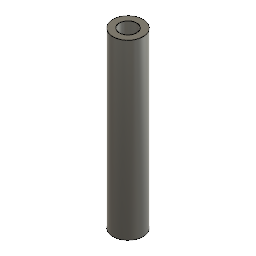
3d (Autodesk Fusion 360 archive; units mm, degrees)
design "mount_pole"
Autodesk Fusion 360 part; units mm, degrees
note: some values were not read from the file. Chosen so that the rebuilt part matches the saved one: which face or edge a step refers to.
sketch "Sketch1" plane through (0, 0, 0) normal (0, 1, 0) x (1, 0, 0)
  circle A0 centre (0, 0) radius 3.5
  circle A1 centre (0, 0) radius 2
  dimension "d1" = 7
  dimension "d2" = 4
  measures "d1" diameter of A0
  measures "d2" diameter of A1
extrude "Extrude1" add sketch "Sketch1" along normal blind 40

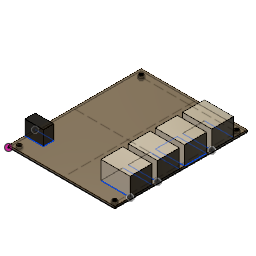
design "ZodiacFX"
Autodesk Fusion 360 part; units mm, degrees
sketch "Sketch1" plane through (0, 0, 0) normal (0, 1, 0) x (1, 0, 0)
  line L0 (0, 0) -> (80, 0)
  line L1 (80, 0) -> (80, 100)
  line L2 (80, 100) -> (0, 100)
  line L3 (0, 100) -> (0, 0)
  circle A0 centre (4, 96) radius 1.5
  circle A1 centre (76, 96) radius 1.5
  circle A2 centre (76, 4) radius 1.5
  circle A3 centre (4, 4) radius 1.5
  line L4 (40, 100) -> (40, 0) construction
  line L5 (0, 50) -> (80, 50) construction
  line L6 (4, 96) -> (40, 96) construction
  line L7 (76, 96) -> (76, 50) construction
  line L8 (76, 96) -> (40, 96) construction
  line L9 (76, 50) -> (76, 4) construction
  dimension "d1" = 80
  dimension "d2" = 100
  dimension "d3" = 3
  dimension "d4" = 72
  dimension "d5" = 92
  measures "d1" distance of L0.start
  measures "d3" diameter of A0
  measures "d5" distance of L0.start
extrude "Extrude1" add sketch "Sketch1" along normal blind 1.6
sketch "Sketch2" plane through (0, 1.6, 0) normal (0, 1, 0) x (-1, 0, 0)
  circle A0 centre (-4, -96) radius 1.5
  circle A1 centre (-4, -4) radius 1.5
  circle A2 centre (-76, -96) radius 1.5
  circle A3 centre (-76, -4) radius 1.5
  line L0 (0, -100) -> (0, 0)
  line L1 (0, 0) -> (-80, 0)
  line L2 (-80, 0) -> (-80, -100)
  line L3 (-80, -100) -> (0, -100)
  line L4 (-58, -89.6377) -> (-80, -89.6377)
  line L5 (-80, -89.6377) -> (-80, -73.1377)
  line L6 (-80, -73.1377) -> (-58, -73.1377)
  line L7 (-58, -73.1377) -> (-58, -89.6377)
  line L8 (-58, -69.1377) -> (-80, -69.1377)
  line L9 (-80, -69.1377) -> (-80, -52.6377)
  line L10 (-80, -52.6377) -> (-58, -52.6377)
  line L11 (-58, -52.6377) -> (-58, -69.1377)
  line L12 (-58, -48.6377) -> (-80, -48.6377)
  line L13 (-80, -48.6377) -> (-80, -32.1377)
  line L14 (-80, -32.1377) -> (-58, -32.1377)
  line L15 (-58, -32.1377) -> (-58, -48.6377)
  line L16 (-58, -28.1377) -> (-80, -28.1377)
  line L17 (-80, -28.1377) -> (-80, -11.6377)
  line L18 (-80, -11.6377) -> (-58, -11.6377)
  line L19 (-58, -11.6377) -> (-58, -28.1377)
  line L20 (0, -20) -> (-14.1052, -20)
  line L21 (-14.1052, -20) -> (-14.1052, -12.0995)
  line L22 (-14.1052, -12.0995) -> (0, -12.0995)
  line L23 (0, -12.0995) -> (0, -20)
  dimension "d8" = 16.5
  dimension "d9" = 22
  dimension "d10" = 4
  dimension "d11" = 4
  dimension "d12" = 4
  measures "d10" distance of L6 L8
  measures "d11" distance of L10 L12
  measures "d12" distance of L14 L16
extrude "Extrude2" add sketch "Sketch2" along normal blind 13.8 contours L2 L4 L5 L6 L7 | L2 L8 L9 L10 L11 | L2 L16 L17 L18 L19 | L2 L12 L13 L14 L15
extrude "Extrude3" add sketch "Sketch2" along normal blind 11 contours L0 L20 L21 L22 L23
sketch "Sketch3" plane through (0, 1.6, 0) normal (0, 1, 0) x (-1, 0, 0)

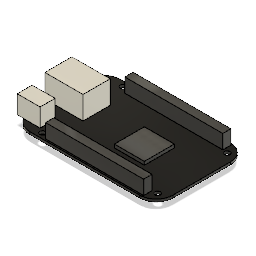
design "BeagleBoneBlack"
Autodesk Fusion 360 part; units mm, degrees
sketch "Sketch1" plane through (0, 0, 0) normal (0, 1, 0) x (1, 0, 0)
  line L0 (10, 0) -> (76.2, 0)
  line L1 (86.2, 10) -> (86.2, 44.61)
  line L2 (76.2, 54.61) -> (10, 54.61)
  line L3 (0, 44.61) -> (0, 10)
  circle A0 centre (14.6, 51.435) radius 1.6
  circle A1 centre (14.6, 3.175) radius 1.6
  circle A2 centre (80.64, 48.26) radius 1.6
  circle A3 centre (80.64, 6.35) radius 1.6
  arc A4 (0, 10) -> (10, 0) centre (10, 10) ccw
  arc A5 (10, 54.61) -> (0, 44.61) centre (10, 44.61) ccw
  arc A6 (86.2, 44.61) -> (76.2, 54.61) centre (76.2, 44.61) ccw
  arc A7 (76.2, 0) -> (86.2, 10) centre (76.2, 10) ccw
  dimension "d1" = 86.2
  dimension "d2" = 54.61
  dimension "d3" = 3.2
  dimension "d4" = 14.6
  dimension "d5" = 3.175
  dimension "d6" = 48.26
  dimension "d8" = 41.91
  dimension "d10" = 6.35
  dimension "d11" = 65.9
  dimension "d12" = 66.04
  dimension "d13" = 10
  dimension "d36" = 3.11
  measures "d1" distance of origin
  measures "d2" distance of origin
  measures "d3" diameter of A1
  measures "d4" distance of L3
  measures "d5" distance of L2
  measures "d8" distance of origin
  measures "d10" distance of L0
  measures "d12" distance of origin
  measures "d13" radius of A4
extrude "Extrude1" add sketch "Sketch1" along normal blind 1.6
sketch "Sketch2" plane through (0, 1.6, 0) normal (0, 1, 0) x (-1, 0, 0)
  circle A0 centre (-14.6, -3.175) radius 1.6
  circle A1 centre (-80.64, -6.35) radius 1.6
  circle A2 centre (-14.6, -51.435) radius 1.6
  circle A3 centre (-80.64, -48.26) radius 1.6
  arc A4 (-76.2, 0) -> (-86.2, -10) centre (-76.2, -10) ccw
  line L0 (-86.2, -10) -> (-86.2, -44.61)
  arc A5 (-86.2, -44.61) -> (-76.2, -54.61) centre (-76.2, -44.61) ccw
  line L1 (-76.2, -54.61) -> (-10, -54.61)
  arc A6 (-10, -54.61) -> (0, -44.61) centre (-10, -44.61) ccw
  line L2 (0, -44.61) -> (0, -10)
  arc A7 (0, -10) -> (-10, 0) centre (-10, -10) ccw
  line L3 (-10, 0) -> (-76.2, 0)
  line L4 (-18.553, -6) -> (-77.553, -6)
  line L5 (-77.553, -6) -> (-77.553, -1)
  line L6 (-77.553, -1) -> (-18.553, -1)
  line L7 (-18.553, -1) -> (-18.553, -6)
  line L8 (-18.553, -53.61) -> (-77.553, -53.61)
  line L9 (-77.553, -53.61) -> (-77.553, -48.61)
  line L10 (-77.553, -48.61) -> (-18.553, -48.61)
  line L11 (-18.553, -48.61) -> (-18.553, -53.61)
  dimension "d16" = 59
  dimension "d17" = 1
  dimension "d18" = 1
  dimension "d19" = 5
  measures "d16" distance of origin
  measures "d17" distance of L1 L8
  measures "d18" distance of L3 L6
extrude "Extrude2" add sketch "Sketch2" along normal blind 8.5 contours L4 L5 L6 L7 | L8 L9 L10 L11
sketch "Sketch3" plane through (0, 1.6, 0) normal (0, 1, 0) x (-1, 0, 0)
  line L0 (-18.553, -1) -> (-18.553, -6)
  line L1 (-18.553, -6) -> (-77.553, -6)
  line L2 (-77.553, -6) -> (-77.553, -1)
  line L3 (-77.553, -1) -> (-18.553, -1)
  line L4 (-18.553, -48.61) -> (-18.553, -53.61)
  line L5 (-18.553, -53.61) -> (-77.553, -53.61)
  line L6 (-77.553, -53.61) -> (-77.553, -48.61)
  line L7 (-77.553, -48.61) -> (-18.553, -48.61)
  circle A0 centre (-14.6, -3.175) radius 1.6
  circle A1 centre (-80.64, -6.35) radius 1.6
  circle A2 centre (-14.6, -51.435) radius 1.6
  circle A3 centre (-80.64, -48.26) radius 1.6
  arc A4 (-76.2, 0) -> (-86.2, -10) centre (-76.2, -10) ccw
  line L8 (-86.2, -10) -> (-86.2, -44.61)
  arc A5 (-86.2, -44.61) -> (-76.2, -54.61) centre (-76.2, -44.61) ccw
  line L9 (-76.2, -54.61) -> (-10, -54.61)
  arc A6 (-10, -54.61) -> (0, -44.61) centre (-10, -44.61) ccw
  line L10 (0, -44.61) -> (0, -10)
  arc A7 (0, -10) -> (-10, 0) centre (-10, -10) ccw
  line L11 (-10, 0) -> (-76.2, 0)
  line L12 (2.5, -37.91) -> (-20.5, -37.91)
  line L13 (-20.5, -37.91) -> (-20.5, -21.61)
  line L14 (-20.5, -21.61) -> (2.5, -21.61)
  line L15 (2.5, -21.61) -> (2.5, -37.91)
  dimension "d22" = 16.3
  dimension "d23" = 16.7
  dimension "d24" = 2.5
  measures "d23" distance of L9 L12
  measures "d24" distance of L10 L15
extrude "Extrude3" add sketch "Sketch3" along normal blind 13.8 contours L10 L12 L14 L15 | L10 L12 L13 L14
sketch "Sketch4" plane through (0, 1.6, 0) normal (0, 1, 0) x (-1, 0, 0)
  line L0 (-20.5, -21.61) -> (0, -21.61)
  line L1 (0, -21.61) -> (0, -10)
  arc A0 (0, -10) -> (-10, 0) centre (-10, -10) ccw
  line L2 (-10, 0) -> (-76.2, 0)
  arc A1 (-76.2, 0) -> (-86.2, -10) centre (-76.2, -10) ccw
  line L3 (-86.2, -10) -> (-86.2, -44.61)
  arc A2 (-86.2, -44.61) -> (-76.2, -54.61) centre (-76.2, -44.61) ccw
  line L4 (-76.2, -54.61) -> (-10, -54.61)
  arc A3 (-10, -54.61) -> (0, -44.61) centre (-10, -44.61) ccw
  line L5 (0, -44.61) -> (0, -37.91)
  line L6 (0, -37.91) -> (-20.5, -37.91)
  line L7 (-20.5, -37.91) -> (-20.5, -21.61)
  line L8 (-18.553, -1) -> (-18.553, -6)
  line L9 (-18.553, -6) -> (-77.553, -6)
  line L10 (-77.553, -6) -> (-77.553, -1)
  line L11 (-77.553, -1) -> (-18.553, -1)
  line L12 (-18.553, -48.61) -> (-18.553, -53.61)
  line L13 (-18.553, -53.61) -> (-77.553, -53.61)
  line L14 (-77.553, -53.61) -> (-77.553, -48.61)
  line L15 (-77.553, -48.61) -> (-18.553, -48.61)
  circle A4 centre (-14.6, -3.175) radius 1.6
  circle A5 centre (-80.64, -6.35) radius 1.6
  circle A6 centre (-14.6, -51.435) radius 1.6
  circle A7 centre (-80.64, -48.26) radius 1.6
  line L16 (2.5, -14) -> (-11.3258, -14)
  line L17 (-11.3258, -14) -> (-11.3258, -5)
  line L18 (-11.3258, -5) -> (2.5, -5)
  line L19 (2.5, -5) -> (2.5, -14)
  dimension "d27" = 9
  dimension "d28" = 5
  measures "d28" distance of L18
extrude "Extrude4" add sketch "Sketch4" along normal blind 11 contours L1 A0 L16 L17 L18 | L1 A0 L16 L18 L19
sketch "Sketch5" plane through (0, 0, 0) normal (0, -1, 0) x (1, 0, 0)
  circle A0 centre (14.6, -3.175) radius 1.6
  circle A1 centre (80.64, -6.35) radius 1.6
  circle A2 centre (14.6, -51.435) radius 1.6
  circle A3 centre (80.64, -48.26) radius 1.6
  arc A4 (86.2, -10) -> (76.2, 0) centre (76.2, -10) ccw
  line L0 (76.2, 0) -> (10, 0)
  arc A5 (10, 0) -> (0, -10) centre (10, -10) ccw
  line L1 (0, -10) -> (0, -44.61)
  arc A6 (0, -44.61) -> (10, -54.61) centre (10, -44.61) ccw
  line L2 (10, -54.61) -> (76.2, -54.61)
  arc A7 (76.2, -54.61) -> (86.2, -44.61) centre (76.2, -44.61) ccw
  line L3 (86.2, -44.61) -> (86.2, -10)
  line L4 (-0.5891, -40.4049) -> (7.6203, -40.4049)
  line L5 (7.6203, -40.4049) -> (7.6203, -46.4306)
  line L6 (7.6203, -46.4306) -> (-0.5891, -46.4306)
  line L7 (-0.5891, -46.4306) -> (-0.5891, -40.4049)
extrude "Extrude5" add sketch "Sketch5" along normal blind 3.9 contours L1 A6 L4 L5 L6 | L1 A6 L4 L6 L7
sketch "Sketch6" plane through (0, 1.6, 0) normal (0, 1, 0) x (-1, 0, 0)
  line L0 (-11.3258, -5) -> (-1.3397, -5)
  arc A0 (-1.3397, -5) -> (-10, 0) centre (-10, -10) ccw
  line L1 (-10, 0) -> (-76.2, 0)
  arc A1 (-76.2, 0) -> (-86.2, -10) centre (-76.2, -10) ccw
  line L2 (-86.2, -10) -> (-86.2, -44.61)
  arc A2 (-86.2, -44.61) -> (-76.2, -54.61) centre (-76.2, -44.61) ccw
  line L3 (-76.2, -54.61) -> (-10, -54.61)
  arc A3 (-10, -54.61) -> (0, -44.61) centre (-10, -44.61) ccw
  line L4 (0, -44.61) -> (0, -37.91)
  line L5 (0, -37.91) -> (-20.5, -37.91)
  line L6 (-20.5, -37.91) -> (-20.5, -21.61)
  line L7 (-20.5, -21.61) -> (0, -21.61)
  line L8 (0, -21.61) -> (0, -14)
  line L9 (0, -14) -> (-11.3258, -14)
  line L10 (-11.3258, -14) -> (-11.3258, -5)
  line L11 (-18.553, -1) -> (-18.553, -6)
  line L12 (-18.553, -6) -> (-77.553, -6)
  line L13 (-77.553, -6) -> (-77.553, -1)
  line L14 (-77.553, -1) -> (-18.553, -1)
  line L15 (-18.553, -48.61) -> (-18.553, -53.61)
  line L16 (-18.553, -53.61) -> (-77.553, -53.61)
  line L17 (-77.553, -53.61) -> (-77.553, -48.61)
  line L18 (-77.553, -48.61) -> (-18.553, -48.61)
  circle A4 centre (-14.6, -3.175) radius 1.6
  circle A5 centre (-80.64, -6.35) radius 1.6
  circle A6 centre (-14.6, -51.435) radius 1.6
  circle A7 centre (-80.64, -48.26) radius 1.6
  line L19 (-44, -35) -> (-62, -35)
  line L20 (-62, -35) -> (-62, -17)
  line L21 (-62, -17) -> (-44, -17)
  line L22 (-44, -17) -> (-44, -35)
  dimension "d33" = 18
  measures "d33" distance of origin
extrude "Extrude6" add sketch "Sketch6" along normal blind 2 contours L19 L20 L21 L22

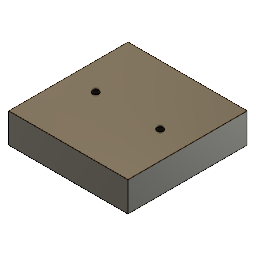
design "switch"
Autodesk Fusion 360 part; units mm, degrees
sketch "Sketch1" plane through (0, 0, 0) normal (0, 1, 0) x (1, 0, 0)
  line L0 (0, 0) -> (0, 100)
  line L1 (0, 100) -> (-100, 100)
  line L2 (-100, 100) -> (-100, 0)
  line L3 (-100, 0) -> (0, 0)
  dimension "d1" = 100
  dimension "d2" = 100
  dimension "d3" = 100
extrude "Extrude1" add sketch "Sketch1" along normal blind 25
sketch "Sketch2" plane through (0, 25, 0) normal (0, 1, 0) x (-1, 0, 0)
  line L0 (100, 0) -> (0, 0)
  line L1 (0, 0) -> (0, -100)
  line L2 (0, -100) -> (100, -100)
  line L3 (100, -100) -> (100, 0)
  circle A0 centre (23, -50) radius 2.5
  circle A1 centre (77, -50) radius 2.5
  dimension "d6" = 5
  dimension "d7" = 5
  dimension "d8" = 23
  dimension "d9" = 23
  dimension "d10" = 50
  dimension "d11" = 50
  dimension "d14" = 54
  measures "d6" diameter of A0
  measures "d7" diameter of A1
extrude "Extrude2" cut sketch "Sketch2" against normal blind 90 contours A0 | A1

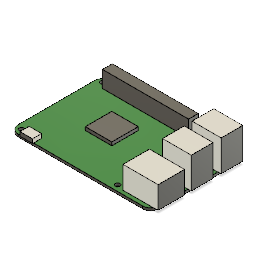
design "RPi"
Autodesk Fusion 360 part; units mm, degrees
sketch "Sketch1" plane through (0, 0, 0) normal (0, 1, 0) x (1, 0, 0)
  line L0 (11.7853, -3.8171) -> (86.7853, -3.8171)
  line L1 (91.7853, -8.8171) -> (91.7853, -54.8171)
  line L2 (86.7853, -59.8171) -> (11.7853, -59.8171)
  line L3 (6.7853, -54.8171) -> (6.7853, -8.8171)
  circle A0 centre (10.2853, -7.3171) radius 1.4
  circle A1 centre (10.2853, -56.3171) radius 1.4
  circle A2 centre (68.2853, -7.3171) radius 1.4
  circle A3 centre (68.2853, -56.3171) radius 1.4
  arc A4 (91.7853, -8.8171) -> (86.7853, -3.8171) centre (86.7853, -8.8171) ccw
  arc A5 (86.7853, -59.8171) -> (91.7853, -54.8171) centre (86.7853, -54.8171) ccw
  arc A6 (6.7853, -54.8171) -> (11.7853, -59.8171) centre (11.7853, -54.8171) ccw
  arc A7 (11.7853, -3.8171) -> (6.7853, -8.8171) centre (11.7853, -8.8171) ccw
  dimension "d1" = 85
  dimension "d2" = 56
  dimension "d3" = 58
  dimension "d4" = 2.8
  dimension "d5" = 3.5
  dimension "d6" = 3.5
  dimension "d7" = 49
  dimension "d8" = 5
  measures "d1" distance of origin
  measures "d2" distance of origin
  measures "d4" diameter of A0
  measures "d5" distance of L3
  measures "d6" distance of L0
  measures "d8" radius of A4
extrude "Extrude1" add sketch "Sketch1" along normal blind 1.6 makes body 1
copy_body "Body->Comp1" bodies 1 removing the originals makes body 2 in component "PCB"
sketch "Sketch1 (2)" plane through (0, 1.6, 0) normal (0, 1, 0) x (-1, 0, 0) in component "Component"
  circle A0 centre (-68.2853, 56.3171) radius 1.4
  circle A1 centre (-68.2853, 7.3171) radius 1.4
  circle A2 centre (-10.2853, 7.3171) radius 1.4
  circle A3 centre (-10.2853, 56.3171) radius 1.4
  arc A4 (-91.7853, 8.8171) -> (-86.7853, 3.8171) centre (-86.7853, 8.8171) ccw
  line L0 (-86.7853, 3.8171) -> (-11.7853, 3.8171)
  arc A5 (-11.7853, 3.8171) -> (-6.7853, 8.8171) centre (-11.7853, 8.8171) ccw
  line L1 (-6.7853, 8.8171) -> (-6.7853, 54.8171)
  arc A6 (-6.7853, 54.8171) -> (-11.7853, 59.8171) centre (-11.7853, 54.8171) ccw
  line L2 (-11.7853, 59.8171) -> (-86.7853, 59.8171)
  arc A7 (-86.7853, 59.8171) -> (-91.7853, 54.8171) centre (-86.7853, 54.8171) ccw
  line L3 (-91.7853, 54.8171) -> (-91.7853, 8.8171)
  line L4 (-72.7561, 41.6171) -> (-93.8853, 41.6171)
  line L5 (-93.8853, 41.6171) -> (-93.8853, 57.5171)
  line L6 (-93.8853, 57.5171) -> (-72.7561, 57.5171)
  line L7 (-72.7561, 57.5171) -> (-72.7561, 41.6171)
  dimension "d11" = 15.9
  dimension "d12" = 2.3
  dimension "d13" = 87.1
  measures "d12" distance of L2 L6
  measures "d13" distance of L1 L5
extrude "Extrude1'" add sketch "Sketch1 (2)" along normal blind 13.5 contours A7 L3 L4 L5 L6 | A7 L3 L4 L6 L7 bodies 2 in component "PCB"
sketch "Sketch2" plane through (0, 1.6, 0) normal (0, 1, 0) x (-1, 0, 0)
  line L0 (-72.7561, 41.6171) -> (-91.7853, 41.6171)
  line L1 (-91.7853, 41.6171) -> (-91.7853, 8.8171)
  arc A0 (-91.7853, 8.8171) -> (-86.7853, 3.8171) centre (-86.7853, 8.8171) ccw
  line L2 (-86.7853, 3.8171) -> (-11.7853, 3.8171)
  arc A1 (-11.7853, 3.8171) -> (-6.7853, 8.8171) centre (-11.7853, 8.8171) ccw
  line L3 (-6.7853, 8.8171) -> (-6.7853, 54.8171)
  arc A2 (-6.7853, 54.8171) -> (-11.7853, 59.8171) centre (-11.7853, 54.8171) ccw
  line L4 (-11.7853, 59.8171) -> (-86.7853, 59.8171)
  arc A3 (-86.7853, 59.8171) -> (-90.9936, 57.5171) centre (-86.7853, 54.8171) ccw
  line L5 (-90.9936, 57.5171) -> (-72.7561, 57.5171)
  line L6 (-72.7561, 57.5171) -> (-72.7561, 41.6171)
  circle A4 centre (-68.2853, 56.3171) radius 1.4
  circle A5 centre (-68.2853, 7.3171) radius 1.4
  circle A6 centre (-10.2853, 56.3171) radius 1.4
  circle A7 centre (-10.2853, 7.3171) radius 1.4
  line L7 (-13.5853, 55) -> (-21.0853, 55)
  line L8 (-21.0853, 55) -> (-21.0853, 60.4415)
  line L9 (-21.0853, 60.4415) -> (-13.5853, 60.4415)
  line L10 (-13.5853, 60.4415) -> (-13.5853, 55)
  dimension "d16" = 7.5
  dimension "d17" = 6.8
  measures "d16" distance of origin
  measures "d17" distance of L3
extrude "Extrude2" add sketch "Sketch2" along normal blind 2.5 contours L4 L8 L9 L10 | L4 L7 L8 L10 bodies 2 in component "PCB"
sketch "Sketch3" plane through (0, 1.6, 0) normal (0, 1, 0) x (-1, 0, 0)
  line L0 (-21.0853, 55) -> (-21.0853, 59.8171)
  line L1 (-21.0853, 59.8171) -> (-86.7853, 59.8171)
  arc A0 (-86.7853, 59.8171) -> (-90.9936, 57.5171) centre (-86.7853, 54.8171) ccw
  line L2 (-90.9936, 57.5171) -> (-72.7561, 57.5171)
  line L3 (-72.7561, 57.5171) -> (-72.7561, 41.6171)
  line L4 (-72.7561, 41.6171) -> (-91.7853, 41.6171)
  line L5 (-91.7853, 41.6171) -> (-91.7853, 8.8171)
  arc A1 (-91.7853, 8.8171) -> (-86.7853, 3.8171) centre (-86.7853, 8.8171) ccw
  line L6 (-86.7853, 3.8171) -> (-11.7853, 3.8171)
  arc A2 (-11.7853, 3.8171) -> (-6.7853, 8.8171) centre (-11.7853, 8.8171) ccw
  line L7 (-6.7853, 8.8171) -> (-6.7853, 54.8171)
  arc A3 (-6.7853, 54.8171) -> (-11.7853, 59.8171) centre (-11.7853, 54.8171) ccw
  line L8 (-11.7853, 59.8171) -> (-13.5853, 59.8171)
  line L9 (-13.5853, 59.8171) -> (-13.5853, 55)
  line L10 (-13.5853, 55) -> (-21.0853, 55)
  circle A4 centre (-68.2853, 56.3171) radius 1.4
  circle A5 centre (-68.2853, 7.3171) radius 1.4
  circle A6 centre (-10.2853, 56.3171) radius 1.4
  circle A7 centre (-10.2853, 7.3171) radius 1.4
  line L11 (-13.3683, 4.6362) -> (-65.3683, 4.6362)
  line L12 (-65.3683, 4.6362) -> (-65.3683, 10.6362)
  line L13 (-65.3683, 10.6362) -> (-13.3683, 10.6362)
  line L14 (-13.3683, 10.6362) -> (-13.3683, 4.6362)
  dimension "d20" = 52
  dimension "d21" = 6
  measures "d21" distance of L11 L13
extrude "Extrude3" add sketch "Sketch3" along normal blind 10 contours L11 L12 L13 L14 bodies 2 in component "PCB"
sketch "Sketch4" plane through (0, 1.6, 0) normal (0, 1, 0) x (-1, 0, 0)
  line L0 (-13.3683, 10.6362) -> (-13.3683, 4.6362)
  line L1 (-13.3683, 4.6362) -> (-65.3683, 4.6362)
  line L2 (-65.3683, 4.6362) -> (-65.3683, 10.6362)
  line L3 (-65.3683, 10.6362) -> (-13.3683, 10.6362)
  line L4 (-21.0853, 55) -> (-21.0853, 59.8171)
  line L5 (-21.0853, 59.8171) -> (-86.7853, 59.8171)
  arc A0 (-86.7853, 59.8171) -> (-90.9936, 57.5171) centre (-86.7853, 54.8171) ccw
  line L6 (-90.9936, 57.5171) -> (-72.7561, 57.5171)
  line L7 (-72.7561, 57.5171) -> (-72.7561, 41.6171)
  line L8 (-72.7561, 41.6171) -> (-91.7853, 41.6171)
  line L9 (-91.7853, 41.6171) -> (-91.7853, 8.8171)
  arc A1 (-91.7853, 8.8171) -> (-86.7853, 3.8171) centre (-86.7853, 8.8171) ccw
  line L10 (-86.7853, 3.8171) -> (-11.7853, 3.8171)
  arc A2 (-11.7853, 3.8171) -> (-6.7853, 8.8171) centre (-11.7853, 8.8171) ccw
  line L11 (-6.7853, 8.8171) -> (-6.7853, 54.8171)
  arc A3 (-6.7853, 54.8171) -> (-11.7853, 59.8171) centre (-11.7853, 54.8171) ccw
  line L12 (-11.7853, 59.8171) -> (-13.5853, 59.8171)
  line L13 (-13.5853, 59.8171) -> (-13.5853, 55)
  line L14 (-13.5853, 55) -> (-21.0853, 55)
  circle A4 centre (-68.2853, 56.3171) radius 1.4
  circle A5 centre (-68.2853, 7.3171) radius 1.4
  circle A6 centre (-10.2853, 56.3171) radius 1.4
  circle A7 centre (-10.2853, 7.3171) radius 1.4
  line L15 (-30.1471, 21.6994) -> (-46.1471, 21.6994)
  line L16 (-46.1471, 21.6994) -> (-46.1471, 37.6994)
  line L17 (-46.1471, 37.6994) -> (-30.1471, 37.6994)
  line L18 (-30.1471, 37.6994) -> (-30.1471, 21.6994)
  dimension "d24" = 16
  dimension "d25" = 16
extrude "Extrude4" add sketch "Sketch4" along normal blind 2 contours L15 L16 L17 L18 bodies 2 in component "PCB"
sketch "Sketch5" plane through (0, 1.6, 0) normal (0, 1, 0) x (-1, 0, 0)
  line L0 (-30.1471, 37.6994) -> (-30.1471, 21.6994)
  line L1 (-30.1471, 21.6994) -> (-46.1471, 21.6994)
  line L2 (-46.1471, 21.6994) -> (-46.1471, 37.6994)
  line L3 (-46.1471, 37.6994) -> (-30.1471, 37.6994)
  line L4 (-13.3683, 10.6362) -> (-13.3683, 4.6362)
  line L5 (-13.3683, 4.6362) -> (-65.3683, 4.6362)
  line L6 (-65.3683, 4.6362) -> (-65.3683, 10.6362)
  line L7 (-65.3683, 10.6362) -> (-13.3683, 10.6362)
  line L8 (-21.0853, 55) -> (-21.0853, 59.8171)
  line L9 (-21.0853, 59.8171) -> (-86.7853, 59.8171)
  arc A0 (-86.7853, 59.8171) -> (-90.9936, 57.5171) centre (-86.7853, 54.8171) ccw
  line L10 (-90.9936, 57.5171) -> (-72.7561, 57.5171)
  line L11 (-72.7561, 57.5171) -> (-72.7561, 41.6171)
  line L12 (-72.7561, 41.6171) -> (-91.7853, 41.6171)
  line L13 (-91.7853, 41.6171) -> (-91.7853, 8.8171)
  arc A1 (-91.7853, 8.8171) -> (-86.7853, 3.8171) centre (-86.7853, 8.8171) ccw
  line L14 (-86.7853, 3.8171) -> (-11.7853, 3.8171)
  arc A2 (-11.7853, 3.8171) -> (-6.7853, 8.8171) centre (-11.7853, 8.8171) ccw
  line L15 (-6.7853, 8.8171) -> (-6.7853, 54.8171)
  arc A3 (-6.7853, 54.8171) -> (-11.7853, 59.8171) centre (-11.7853, 54.8171) ccw
  line L16 (-11.7853, 59.8171) -> (-13.5853, 59.8171)
  line L17 (-13.5853, 59.8171) -> (-13.5853, 55)
  line L18 (-13.5853, 55) -> (-21.0853, 55)
  circle A4 centre (-68.2853, 56.3171) radius 1.4
  circle A5 centre (-68.2853, 7.3171) radius 1.4
  circle A6 centre (-10.2853, 56.3171) radius 1.4
  circle A7 centre (-10.2853, 7.3171) radius 1.4
  line L19 (-76.4643, 24.3171) -> (-93.7853, 24.3171)
  line L20 (-93.7853, 24.3171) -> (-93.7853, 37.4171)
  line L21 (-93.7853, 37.4171) -> (-76.4643, 37.4171)
  line L22 (-76.4643, 37.4171) -> (-76.4643, 24.3171)
  line L23 (-76.2496, 19.4171) -> (-93.7853, 19.4171)
  line L24 (-93.7853, 19.4171) -> (-93.7853, 6.3171)
  line L25 (-93.7853, 6.3171) -> (-76.2496, 6.3171)
  line L26 (-76.2496, 6.3171) -> (-76.2496, 19.4171)
  dimension "d28" = 13.1
  dimension "d29" = 4.2
  dimension "d30" = 2
  dimension "d31" = 13.1
  dimension "d32" = 4.9
  measures "d29" distance of L12 L21
  measures "d30" distance of L13 L20
  measures "d32" distance of L19 L23
extrude "Extrude5" add sketch "Sketch5" along normal blind 18.8 contours L13 L19 L21 L22 | L13 L19 L20 L21 | L13 A1 L23 L24 L25 | L13 A1 L23 L25 L26 bodies 2 in component "PCB"
component "Component" placed x (1, 0, 0) y (0, 1, 0) z (0, 0, 1) at (0, 0, 0)
component "PCB" placed x (1, 0, 0) y (0, 1, 0) z (0, 0, 1) at (0, 0, 0)

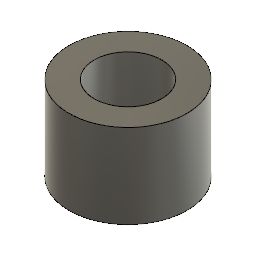
design "comp_pole"
Autodesk Fusion 360 part; units mm, degrees
sketch "Sketch1" plane through (0, 0, 0) normal (0, 1, 0) x (1, 0, 0)
  circle A0 centre (0, 0) radius 3.5
  circle A1 centre (0, 0) radius 2
  dimension "d1" = 7
  dimension "d2" = 4
  measures "d1" diameter of A0
  measures "d2" diameter of A1
extrude "Extrude1" add sketch "Sketch1" along normal blind 5

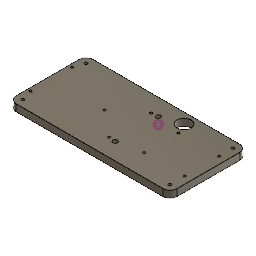
design "botenplata"
Autodesk Fusion 360 part; units mm, degrees
sketch "Sketch2" plane through (0, 0, 0) normal (0, 1, 0) x (1, 0, 0)
  line L0 (0, 0) -> (0, 110)
  line L1 (0, 0) -> (-230, 0)
  line L2 (-230, 0) -> (-230, 110)
  line L3 (-230, 110) -> (0, 110)
  dimension "d30" = 110
  dimension "d31" = 230
  dimension "d32" = 110
  measures "d31" distance of L0.start
  measures "d32" distance of L0.start
extrude "Extrude2" add sketch "Sketch2" along normal blind 10
sketch "Sketch3" plane through (0, 10, 0) normal (0, 1, 0) x (-1, 0, 0)
  line L0 (0, 0) -> (0, -110)
  line L1 (0, -110) -> (230, -110)
  line L2 (230, -110) -> (230, 0)
  line L3 (230, 0) -> (0, 0)
  circle A0 centre (102.5, -24.25) radius 3.25
  circle A1 centre (102.5, -85.75) radius 3.25
  dimension "d35" = 6.5
  dimension "d36" = 102.5
  dimension "d37" = 24.25
  dimension "d91" = 6.5
  dimension "d92" = 61.5
  measures "d35" diameter of A0
  measures "d37" distance of L3 L0.start
  measures "d91" diameter of A1
extrude "Extrude10" cut sketch "Sketch3" against normal blind 25 contours A1
extrude "Extrude3" cut sketch "Sketch3" against normal blind 50 contours A0
ref_plane "WorkPlane3" through (-115, 5, -55) normal (0, 0, 1) x (1, 0, 0)
fillet "Fillet1" radius 10 1 edges at (-230, 5, 0)
fillet "Fillet2" radius 10 3 edges at (-230, 5, -110) (0, 5, 0) (0, 5, -110)
sketch "Sketch4" plane through (0, 10, 0) normal (0, 1, 0) x (-1, 0, 0)
  arc A0 (0, -100) -> (10, -110) centre (10, -100) ccw
  line L0 (10, -110) -> (220, -110)
  arc A1 (220, -110) -> (230, -100) centre (220, -100) ccw
  line L1 (230, -100) -> (230, -10)
  arc A2 (230, -10) -> (220, 0) centre (220, -10) ccw
  line L2 (220, 0) -> (10, 0)
  arc A3 (10, 0) -> (0, -10) centre (10, -10) ccw
  line L3 (0, -10) -> (0, -100)
  circle A4 centre (102.5, -24.25) radius 3.25
  circle A5 centre (75, -95) radius 10
  circle A6 centre (102.5, -85.75) radius 3.25
  dimension "d44" = 20
  dimension "d90" = 3.5
  measures "d44" diameter of A5
extrude "Extrude4" cut sketch "Sketch4" against normal blind 45 contours A5
sketch "Sketch5" plane through (0, 10, 0) normal (0, 1, 0) x (-1, 0, 0)
  circle A0 centre (75, -95) radius 10
  arc A1 (0, -100) -> (10, -110) centre (10, -100) ccw
  line L0 (10, -110) -> (220, -110)
  arc A2 (220, -110) -> (230, -100) centre (220, -100) ccw
  line L1 (230, -100) -> (230, -10)
  arc A3 (230, -10) -> (220, 0) centre (220, -10) ccw
  line L2 (220, 0) -> (10, 0)
  arc A4 (10, 0) -> (0, -10) centre (10, -10) ccw
  line L3 (0, -10) -> (0, -100)
  circle A5 centre (102.5, -24.25) radius 3.25
  circle A6 centre (220, -100) radius 2
  circle A7 centre (102.5, -85.75) radius 3.25
  dimension "d47" = 4
  measures "d47" diameter of A6
extrude "Extrude5" cut sketch "Sketch5" against normal blind 23 contours A6
pattern_linear "R-Pattern1" count 2 spacing 90 along (0, 0, 1) of "Extrude5"
pattern_linear "R-Pattern2" count 2 spacing 210 along (1, 0, 0) of 2 faces at (-221.8794, 3.3333, -99.316) (-219.0876, 6.6667, -11.7797)
sketch "Sketch7" plane through (0, 10, 0) normal (0, 1, 0) x (-1, 0, 0)
  circle A0 centre (10, -80) radius 1.75
  circle A1 centre (10, -31) radius 1.75
  circle A2 centre (68, -31) radius 1.75
  circle A3 centre (68, -80) radius 1.75
  dimension "d58" = 3.5
  dimension "d59" = 3.5
  dimension "d60" = 3.5
  dimension "d61" = 3.5
  dimension "d62" = 49
  dimension "d63" = 58
  dimension "d64" = 58
  dimension "d65" = 49
  measures "d58" diameter of A0
  measures "d59" diameter of A1
  measures "d60" diameter of A2
  measures "d61" diameter of A3
  measures "d63" distance of origin
  measures "d64" distance of origin
sketch "Sketch8" plane through (0, 10, 0) normal (0, 1, 0) x (-1, 0, 0)
  circle A0 centre (10, -10) radius 2
  circle A1 centre (10, -100) radius 2
  circle A2 centre (220, -10) radius 2
  circle A3 centre (220, -100) radius 2
  circle A4 centre (75, -95) radius 10
  arc A5 (0, -100) -> (10, -110) centre (10, -100) ccw
  line L0 (10, -110) -> (220, -110)
  arc A6 (220, -110) -> (230, -100) centre (220, -100) ccw
  line L1 (230, -100) -> (230, -10)
  arc A7 (230, -10) -> (220, 0) centre (220, -10) ccw
  line L2 (220, 0) -> (10, 0)
  arc A8 (10, 0) -> (0, -10) centre (10, -10) ccw
  line L3 (0, -10) -> (0, -100)
  circle A9 centre (102.5, -24.25) radius 3.25
  circle A10 centre (225, -85) radius 1.75
  circle A11 centre (225.0348, -26) radius 1.75
  circle A12 centre (112, -85) radius 1.75
  circle A13 centre (112.0348, -25) radius 1.75
  circle A14 centre (102.5, -85.75) radius 3.25
  dimension "d70" = 3.5
  dimension "d71" = 3.5
  dimension "d72" = 59
  dimension "d75" = 3.5
  dimension "d76" = 113
  dimension "d77" = 3.5
  dimension "d78" = 113
  measures "d70" diameter of A10
  measures "d71" diameter of A11
  measures "d75" diameter of A12
  measures "d77" diameter of A13
extrude "Extrude7" cut sketch "Sketch8" against normal blind 40 contours A10 | A11 | A12 | A13
extrude "Extrude8" cut sketch "Sketch7" against normal blind 30
sketch "Sketch9" plane through (0, 10, 0) normal (0, 1, 0) x (-1, 0, 0)
  circle A0 centre (10, -80) radius 1.75
  circle A1 centre (68, -31) radius 1.75
  circle A2 centre (68, -80) radius 1.75
  circle A3 centre (10, -31) radius 1.75
  circle A4 centre (225.0348, -26) radius 1.75
  circle A5 centre (112.0348, -25) radius 1.75
  circle A6 centre (225, -85) radius 1.75
  circle A7 centre (112, -85) radius 1.75
  circle A8 centre (10, -10) radius 2
  circle A9 centre (10, -100) radius 2
  circle A10 centre (220, -10) radius 2
  circle A11 centre (220, -100) radius 2
  circle A12 centre (75, -95) radius 10
  arc A13 (0, -100) -> (10, -110) centre (10, -100) ccw
  line L0 (10, -110) -> (220, -110)
  arc A14 (220, -110) -> (230, -100) centre (220, -100) ccw
  line L1 (230, -100) -> (230, -10)
  arc A15 (230, -10) -> (220, 0) centre (220, -10) ccw
  line L2 (220, 0) -> (10, 0)
  arc A16 (10, 0) -> (0, -10) centre (10, -10) ccw
  line L3 (0, -10) -> (0, -100)
  circle A17 centre (102.5, -24.25) radius 3.25
  circle A18 centre (102.5, -85.75) radius 3.25
sketch "Sketch10" plane through (0, 10, 0) normal (0, 1, 0) x (-1, 0, 0)
  circle A0 centre (149, -55.5) radius 1.75
  circle A1 centre (225.0348, -26) radius 1.75
  dimension "d83" = 3.5
  dimension "d84" = 76
  dimension "d85" = 29.5
  dimension "d86" = 30
  measures "d83" diameter of A0
extrude "Extrude9" cut sketch "Sketch10" against normal blind 55 contours A0
sketch "Sketch11" plane through (0, 10, 0) normal (0, 1, 0) x (-1, 0, 0)
  circle A0 centre (149, -55.5) radius 1.75
  circle A1 centre (10, -80) radius 1.75
  circle A2 centre (68, -31) radius 1.75
  circle A3 centre (68, -80) radius 1.75
  circle A4 centre (10, -31) radius 1.75
  circle A5 centre (225.0348, -26) radius 1.75
  circle A6 centre (112.0348, -25) radius 1.75
  circle A7 centre (225, -85) radius 1.75
  circle A8 centre (112, -85) radius 1.75
  circle A9 centre (10, -10) radius 2
  circle A10 centre (10, -100) radius 2
  circle A11 centre (220, -10) radius 2
  circle A12 centre (220, -100) radius 2
  circle A13 centre (75, -95) radius 10
  arc A14 (0, -100) -> (10, -110) centre (10, -100) ccw
  line L0 (10, -110) -> (220, -110)
  arc A15 (220, -110) -> (230, -100) centre (220, -100) ccw
  line L1 (230, -100) -> (230, -10)
  arc A16 (230, -10) -> (220, 0) centre (220, -10) ccw
  line L2 (220, 0) -> (10, 0)
  arc A17 (10, 0) -> (0, -10) centre (10, -10) ccw
  line L3 (0, -10) -> (0, -100)
  circle A18 centre (102.5, -24.25) radius 3.25
  circle A19 centre (102.5, -85.75) radius 3.25
sketch "Sketch12" plane through (0, 0, 0) normal (0, -1, 0) x (1, 0, 0)
  circle A0 centre (-149, -55.5) radius 1.75
  circle A1 centre (-10, -80) radius 1.75
  circle A2 centre (-68, -31) radius 1.75
  circle A3 centre (-68, -80) radius 1.75
  circle A4 centre (-10, -31) radius 1.75
  circle A5 centre (-225.0348, -26) radius 1.75
  circle A6 centre (-112.0348, -25) radius 1.75
  circle A7 centre (-225, -85) radius 1.75
  circle A8 centre (-112, -85) radius 1.75
  circle A9 centre (-10, -100) radius 2
  circle A10 centre (-10, -10) radius 2
  circle A11 centre (-220, -10) radius 2
  circle A12 centre (-220, -100) radius 2
  circle A13 centre (-75, -95) radius 10
  circle A14 centre (-102.5, -24.25) radius 3.25
  arc A15 (-10, -110) -> (0, -100) centre (-10, -100) ccw
  line L0 (0, -100) -> (0, -10)
  arc A16 (0, -10) -> (-10, 0) centre (-10, -10) ccw
  line L1 (-10, 0) -> (-220, 0)
  arc A17 (-220, 0) -> (-230, -10) centre (-220, -10) ccw
  line L2 (-230, -10) -> (-230, -100)
  arc A18 (-230, -100) -> (-220, -110) centre (-220, -100) ccw
  line L3 (-220, -110) -> (-10, -110)
  circle A19 centre (-102.5, -85.75) radius 3.25
extrude "Extrude6" [suppressed]
extrude "Extrude1" [suppressed]
ref_plane "WorkPlane1" through (-130, 5, -55) normal (0, 0, 1) x (1, 0, 0)
mirror "Mirror1" [suppressed]
ref_plane "WorkPlane2" through (-130, 5, -55) normal (1, 0, 0) x (0, 0, -1)
mirror "Mirror2" [suppressed]

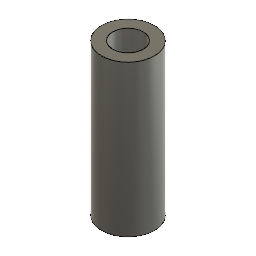
design "fx_mount"
Autodesk Fusion 360 part; units mm, degrees
sketch "Sketch1" plane through (0, 0, 0) normal (0, 1, 0) x (1, 0, 0)
  circle A0 centre (0, 0) radius 3.5
  circle A1 centre (0, 0) radius 2
  dimension "d1" = 7
  dimension "d2" = 4
  measures "d1" diameter of A0
  measures "d2" diameter of A1
extrude "Extrude1" add sketch "Sketch1" along normal blind 20
